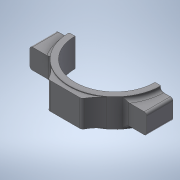
# Autodesk Inventor part: BIELA PART2
Saved by Autodesk Inventor 2020 (Build 240168000, 168)
## iProperties
Created: 2017-10-06
Part Number: BIELA PART2
Material: Generic
Document SubType Name: Modeling
Designer: Usuario
Density: 1 g/cm^3
Appearance: Default
Author: Usuario
Autodesk Inventor part; units mm, degrees
ref_plane "XY Plane" through (0, 0, 0) normal (0, 0, 1) x (1, 0, 0)
sketch "Sketch1" plane through (0, 0, 0) normal (0, 0, 1) x (1, 0, 0)
  arc A0 (-27.5, 0) -> (27.5, 0) centre (0, 0) ccw
  arc A1 (-22.5, 0) -> (22.5, 0) centre (0, 0) ccw
  line L0 (-27.5, 0) -> (-22.5, 0)
  line L1 (22.5, 0) -> (27.5, 0)
  dimension "d0" = 55
  dimension "d1" = 45
  constraints: 4 end point, 4 point on circle, 2 centre point, 2 coincident, 2 horizontal
  measures "d0" diameter of A0
  measures "d1" diameter of A1
extrude "Extrusion1" add sketch "Sketch1" along normal blind 20
ref_plane "Work Plane1" through (-35, 0, 0) normal (1, 0, 0) x (0, 1, 0)
sketch "Sketch2" plane through (-35, 0, 0) normal (1, 0, 0) x (0, 1, 0)
  point P0 (0, 0)
sketch "Sketch3" plane through (-35, 0, 0) normal (1, 0, 0) x (0, 1, 0)
  line L0 (0, 0) -> (0, 20) projected
  line L1 (0, 20) -> (-27.5, 20) projected
sketch "Sketch4" plane through (-35, 0, 0) normal (1, 0, 0) x (0, 1, 0)
  line L0 (0, 4) -> (-16, 4)
  line L1 (-16, 4) -> (-16, 16)
  line L2 (-16, 16) -> (0, 16)
  line L3 (0, 16) -> (0, 4)
  line L4 (0, 0) -> (-27.5, 0) projected
  line L5 (0, 0) -> (0, 10)
  dimension "d5" = 16
  dimension "d6" = 12
  dimension "d7" = 10
  dimension "d8" = 6
  constraints: 10 end point, 2 parallel, 1 collinear, 1 horizontal, 1 midpoint, 1 perpendicular
  measures "d5" distance of L1.end L2.end
  measures "d6" distance of L0.end L1.end
  measures "d7" distance of L4.start L5.end
  measures "d8" distance of L5.end L2.end
extrude "Extrusion2" add sketch "Sketch4" along normal up to next
mirror "Mirror1" about plane through (0, 0, 0) normal (1, 0, 0) of "Extrusion2"
ref_plane "Work Plane2" through (0, -30, 0) normal (0, 1, 0) x (-1, 0, 0)
sketch "Sketch5" plane through (0, -30, 0) normal (0, 1, 0) x (-1, 0, 0)
  line L0 (0, 0) -> (0, 10)
  line L1 (10, 18) -> (-10, 18)
  line L2 (-10, 18) -> (-10, 2)
  line L3 (-10, 2) -> (10, 2)
  line L4 (10, 2) -> (10, 18)
  line L5 (10, 18) -> (-10, 2) construction
  line L6 (-10, 18) -> (10, 2) construction
  dimension "d12" = 10
  dimension "d13" = 20
  dimension "d14" = 16
  constraints: 14 end point, 2 midpoint, 2 parallel, 1 horizontal, 1 perpendicular, 1 vertical
  measures "d12" distance of L0.start L0.end
  measures "d13" distance of L3.end L2.end
  measures "d14" distance of L2.end L1.end
extrude "Extrusion3" add sketch "Sketch5" along normal up to next
fillet "Fillet1" radius 25 2 edges at (10, -25.6174, 10) (-10, -25.6174, 10)
fillet "Fillet2" radius 1.5 4 edges at (-35, -8, 16) (-35, -8, 4) (35, -8, 16) (35, -8, 4)
fillet "Fillet3" radius 3 2 edges at (-22.3663, -16, 10) (22.3663, -16, 10)
fillet "Fillet4" radius 2 2 edges at (10, -30, 10) (-10, -30, 10)
fillet "Fillet5" radius 1 2 edges at (0, -27.5, 20) (0, -27.5, 0)
fillet "Fillet6" radius 2 8 edges at (-21.9465, -16.5711, 4) (-26.1851, -8.4017, 4) (-26.1851, -8.4017, 16) (-21.9465, -16.5711, 16) (26.1851, -8.4017, 16) (21.9465, -16.5711, 16) (21.9465, -16.5711, 4) (26.1851, -8.4017, 4)
chamfer "Chamfer1" distance 1 angle 45 2 edges at (0, -22.5, 20) (0, -22.5, 0)
fillet "Fillet7" radius 0.5 26 edges at (-27.2071, 0, 19.7071) (-27.5, 0, 18.5) (-28.0858, 0, 16.5858) (-31.5, 0, 16) (-34.5607, 0, 15.5607) (-35, 0, 10) (-34.5607, 0, 4.4393) (-31.5, 0, 4) (-28.0858, 0, 3.4142) (-27.5, 0, 1.5) (-27.2071, 0, 0.2929) (-25, 0, 0) (-25, 0, 20) (25, 0, 20) (27.5, 0, 18.5) (28.0858, 0, 16.5858) (31.5, 0, 16) (34.5607, 0, 15.5607) (35, 0, 10) (34.5607, 0, 4.4393) (31.5, 0, 4) (28.0858, 0, 3.4142) (27.5, 0, 1.5) (27.2071, 0, 0.2929) (25, 0, 0) (27.2071, 0, 19.7071)
scale "Scale1" factors (0.24, 0.24, 0.24) then translate (0, 0, 7.6) bodies 1
sketch "Sketch8" plane through (0, 0, 12.4) normal (0, 0, 1) x (1, 0, 0)
  circle A0 centre (0, 0) radius 5.75
  dimension "d38" = 11.5
  constraints: 1 centre point, 1 coincident
  measures "d38" diameter of A0
extrude "Extrusion6" cut sketch "Sketch8" against normal blind 10
sketch "Sketch9" plane through (-2.1149, -7.2, 8.08) normal (0, -1, 0) x (1, 0, 0)
  line L0 (0, -0.12) -> (-5.5652, -0.12)
  line L1 (-5.5652, -0.12) -> (9.5234, -0.12)
  line L2 (9.5234, -0.12) -> (9.5234, -1.3413)
  line L3 (9.5234, -1.3413) -> (-5.5652, -1.3413)
  line L4 (-5.5652, -1.3413) -> (-5.5652, -0.12)
  line L5 (0, 3.9481) -> (-5.5652, 3.9481)
  line L6 (-5.5652, 3.9481) -> (9.629, 3.9481)
  line L7 (9.629, 3.9481) -> (9.629, 4.8977)
  line L8 (9.629, 4.8977) -> (-5.5652, 4.8977)
  line L9 (-5.5652, 4.8977) -> (-5.5652, 3.9481)
  point P0 (2.1149, -8.08)
  constraints: 20 end point, 4 horizontal, 4 parallel, 2 perpendicular
extrude "Extrusion7" cut sketch "Sketch9" against normal blind 10
body "Solid1"
